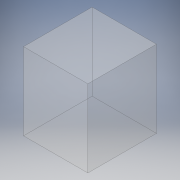
# Autodesk Inventor part: Tall Build Volume
Saved by Autodesk Inventor 2017 (Build 210142000, 142)
## iProperties
Created: 2017-01-10
Part Number: Tall Build Volume
Material: Generic
Document SubType Name: Modeling
Designer: Roksbot
Density: 1 g/cm^3
Appearance: Polycarbonate - Clear
Author: Roksbot
Autodesk Inventor part; units mm, degrees
ref_plane "YZ Plane" through (0, 0, 0) normal (1, 0, 0) x (0, 1, 0)
ref_plane "XZ Plane" through (0, 0, 0) normal (0, 1, 0) x (-1, 0, 0)
ref_plane "XY Plane" through (0, 0, 0) normal (0, 0, 1) x (1, 0, 0)
sketch "Sketch1" plane through (0, 0, 0) normal (0, 1, 0) x (-1, 0, 0)
  line L0 (-381, 406.4) -> (381, 406.4)
  line L1 (381, 406.4) -> (381, -406.4)
  line L2 (381, -406.4) -> (-381, -406.4)
  line L3 (-381, -406.4) -> (-381, 406.4)
  line L4 (-381, 406.4) -> (381, -406.4) construction
  line L5 (381, 406.4) -> (-381, -406.4) construction
  point P0 (0, 0)
  dimension "d0" = 812.8
  dimension "d1" = 762
  constraints: 12 end point, 2 midpoint, 2 parallel, 1 horizontal, 1 perpendicular
  measures "d0" distance of L2.end L0.start
  measures "d1" distance of L1.end L2.end
extrude "Extrusion1" add sketch "Sketch1" along normal blind 914.4
body "Solid1"
